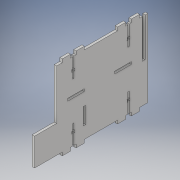
# Autodesk Inventor part: sidewall
Saved by Autodesk Inventor 2018 (Build 220112000, 112)
## iProperties
Created: 2018-03-27
Part Number: sidewall
Material: Generic
Document SubType Name: Modeling
Designer: guita
Density: 1 g/cm^3
Appearance: Default
Author: guita
Autodesk Inventor part; units mm, degrees
ref_plane "YZ Plane" through (0, 0, 0) normal (1, 0, 0) x (0, 1, 0)
ref_plane "XZ Plane" through (0, 0, 0) normal (0, 1, 0) x (-1, 0, 0)
ref_plane "XY Plane" through (0, 0, 0) normal (0, 0, 1) x (1, 0, 0)
sketch "Sketch1" plane through (0, 0, 0) normal (1, 0, 0) x (0, 1, 0)
  line L0 (0, 0) -> (177.8, 0)
  line L1 (177.8, -260.35) -> (0, -260.35)
  line L2 (0, -260.35) -> (0, -241.3)
  line L3 (0, -241.3) -> (-7.62, -241.3)
  line L4 (-7.62, -241.3) -> (-7.62, -222.25)
  line L5 (-7.62, -222.25) -> (0, -222.25)
  line L6 (0, -209.55) -> (-7.62, -209.55)
  line L7 (-7.62, -209.55) -> (-7.62, -190.5)
  line L8 (-7.62, -190.5) -> (0, -190.5)
  line L9 (0, -190.5) -> (0, -152.4)
  line L10 (44.45, -215.9) -> (44.45, -214.2998)
  line L11 (44.45, -217.5002) -> (44.45, -215.9)
  line L12 (24.6348, -214.2998) -> (24.6348, -212.725)
  line L13 (24.6348, -219.075) -> (24.6348, -219.329)
  line L14 (24.6348, -219.329) -> (30.1625, -219.329)
  line L15 (24.6348, -212.725) -> (24.6348, -212.471)
  line L16 (24.6348, -212.471) -> (30.1625, -212.471)
  line L17 (24.6348, -219.075) -> (24.6348, -217.4875)
  line L18 (30.1625, -212.471) -> (30.1625, -214.2998)
  line L19 (30.1625, -217.5002) -> (30.1625, -219.329)
  line L20 (44.45, -214.2998) -> (30.1625, -214.2998)
  line L21 (24.6348, -214.2998) -> (0, -214.2998)
  line L22 (44.45, -217.5002) -> (30.1625, -217.5002)
  line L23 (24.6348, -217.5002) -> (0, -217.5002)
  line L24 (0, -63.5) -> (-7.62, -63.5)
  line L25 (-7.62, -63.5) -> (-7.62, -82.55)
  line L26 (-7.62, -82.55) -> (0, -82.55)
  line L27 (0, -95.25) -> (-7.62, -95.25)
  line L28 (-7.62, -95.25) -> (-7.62, -114.3)
  line L29 (-7.62, -114.3) -> (0, -114.3)
  line L30 (44.45, -88.9) -> (44.45, -90.5002)
  line L31 (44.45, -87.2998) -> (44.45, -88.9)
  line L32 (24.6348, -90.5002) -> (24.6348, -92.075)
  line L33 (24.6348, -85.725) -> (24.6348, -85.471)
  line L34 (24.6348, -85.471) -> (30.1625, -85.471)
  line L35 (24.6348, -92.075) -> (24.6348, -92.329)
  line L36 (24.6348, -92.329) -> (30.1625, -92.329)
  line L37 (24.6348, -85.725) -> (24.6348, -87.3125)
  line L38 (30.1625, -92.329) -> (30.1625, -90.5002)
  line L39 (30.1625, -87.2998) -> (30.1625, -85.471)
  line L40 (44.45, -90.5002) -> (30.1625, -90.5002)
  line L41 (24.6348, -90.5002) -> (0, -90.5002)
  line L42 (44.45, -87.2998) -> (30.1625, -87.2998)
  line L43 (24.6348, -87.2998) -> (0, -87.2998)
  line L44 (177.8, -241.3) -> (185.42, -241.3)
  line L45 (185.42, -241.3) -> (185.42, -222.25)
  line L46 (185.42, -222.25) -> (177.8, -222.25)
  line L47 (177.8, -209.55) -> (185.42, -209.55)
  line L48 (185.42, -209.55) -> (185.42, -190.5)
  line L49 (185.42, -190.5) -> (177.8, -190.5)
  line L50 (177.8, -190.5) -> (177.8, -152.4)
  line L51 (133.35, -215.9) -> (133.35, -214.2998)
  line L52 (133.35, -217.5002) -> (133.35, -215.9)
  line L53 (153.1652, -214.2998) -> (153.1652, -212.725)
  line L54 (153.1652, -219.075) -> (153.1652, -219.329)
  line L55 (153.1652, -219.329) -> (147.6375, -219.329)
  line L56 (153.1652, -212.725) -> (153.1652, -212.471)
  line L57 (153.1652, -212.471) -> (147.6375, -212.471)
  line L58 (153.1652, -219.075) -> (153.1652, -217.4875)
  line L59 (147.6375, -212.471) -> (147.6375, -214.2998)
  line L60 (147.6375, -217.5002) -> (147.6375, -219.329)
  line L61 (133.35, -214.2998) -> (147.6375, -214.2998)
  line L62 (153.1652, -214.2998) -> (177.8, -214.2998)
  line L63 (133.35, -217.5002) -> (147.6375, -217.5002)
  line L64 (153.1652, -217.5002) -> (177.8, -217.5002)
  line L65 (185.42, -63.5) -> (185.42, -82.55)
  line L66 (185.42, -82.55) -> (177.8, -82.55)
  line L67 (177.8, -95.25) -> (185.42, -95.25)
  line L68 (185.42, -95.25) -> (185.42, -114.3)
  line L69 (185.42, -114.3) -> (177.8, -114.3)
  line L70 (153.1652, -85.725) -> (153.1652, -85.471)
  line L71 (153.1652, -85.725) -> (153.1652, -87.3125)
  line L72 (153.1652, -85.471) -> (147.6375, -85.471)
  line L73 (147.6375, -87.2998) -> (147.6375, -85.471)
  line L74 (177.8, -63.5) -> (185.42, -63.5)
  line L75 (153.1652, -90.5002) -> (153.1652, -92.075)
  line L76 (153.1652, -92.075) -> (153.1652, -92.329)
  line L77 (153.1652, -92.329) -> (147.6375, -92.329)
  line L78 (147.6375, -92.329) -> (147.6375, -90.5002)
  line L79 (133.35, -87.2998) -> (147.6375, -87.2998)
  line L80 (133.35, -87.2998) -> (133.35, -88.9)
  line L81 (133.35, -90.5002) -> (147.6375, -90.5002)
  line L82 (153.1652, -87.2998) -> (177.8, -87.2998)
  line L83 (153.1652, -90.5002) -> (177.8, -90.5002)
  line L84 (133.35, -88.9) -> (133.35, -90.5002)
  line L85 (177.8, -260.35) -> (177.8, -254)
  line L86 (177.8, -254) -> (88.9, -254)
  line L87 (88.9, -254) -> (88.9, -247.65)
  line L88 (88.9, -247.65) -> (177.8, -247.65)
  line L89 (177.8, -254) -> (177.8, -260.35)
  line L90 (177.8, 0) -> (177.8, -63.5)
  line L91 (177.8, -114.3) -> (177.8, -190.5)
  line L92 (177.8, -241.3) -> (177.8, -247.65)
  line L93 (0, -260.35) -> (0, -241.3)
  line L94 (0, -190.5) -> (0, -114.3)
  line L95 (0, -63.5) -> (0, 0)
  line L96 (0, -82.55) -> (0, -87.2998)
  line L97 (0, -90.5002) -> (0, -95.25)
  line L98 (0, -95.25) -> (0, -90.5002)
  line L99 (0, -87.2998) -> (0, -82.55)
  line L100 (0, -222.25) -> (0, -217.5002)
  line L101 (0, -214.2998) -> (0, -209.55)
  line L102 (0, -222.25) -> (0, -217.5002)
  line L103 (0, -214.2998) -> (0, -209.55)
  line L104 (177.8, -222.25) -> (177.8, -217.5002)
  line L105 (177.8, -214.2998) -> (177.8, -209.55)
  line L106 (177.8, -209.55) -> (177.8, -214.2998)
  line L107 (177.8, -217.5002) -> (177.8, -222.25)
  line L108 (177.8, -82.55) -> (177.8, -87.2998)
  line L109 (177.8, -90.5002) -> (177.8, -95.25)
  line L110 (177.8, -82.55) -> (177.8, -87.2998)
  line L111 (177.8, -90.5002) -> (177.8, -95.25)
  dimension "d0" = 177.8
  dimension "d1" = 260.35
  dimension "d8" = 38.1
  dimension "d16" = 0.254
  dimension "d17" = 0.254
  dimension "d18" = 6.35
  constraints: 224 end point, 8 point on line, 1 midpoint
  measures "d0" distance of L1.start L1.end
  measures "d1" distance of L0.end L1.start
  measures "d8" distance of L8.end L9.end
  measures "d16" distance of L13.start L13.end
  measures "d17" distance of L12.end L15.end
  measures "d18" distance of L1.start L85.end
extrude "Extrusion1" add sketch "Sketch1" along normal blind 5.5563
sketch "Sketch2" plane through (5.5563, 0, 0) normal (1, 0, 0) x (0, 0, -1)
  line L0 (63.5, 177.8) -> (0, 177.8) projected
  line L1 (0, 177.8) -> (50.8, 177.8)
  line L2 (50.8, 177.8) -> (50.8, 63.5)
  line L3 (50.8, 63.5) -> (0, 63.5)
  line L4 (0, 177.8) -> (0, 0) projected
  line L5 (0, 177.8) -> (0, 63.5)
  constraints: 8 end point, 2 perpendicular, 2 point on line, 1 vertical
extrude "Extrusion2" cut sketch "Sketch2" against normal blind 25.4
sketch "Sketch3" plane through (5.5563, 0, 0) normal (1, 0, 0) x (0, 0, -1)
  line L0 (190.5, 177.8) -> (114.3, 177.8) projected
  line L1 (247.65, 88.9) -> (247.65, 177.8) projected
  line L2 (76.2, 100.8) -> (76.2, 95.25)
  line L3 (114.3, 95.25) -> (114.3, 100.8)
  line L4 (184.15, 100.8) -> (184.15, 95.25)
  line L5 (222.25, 95.25) -> (222.25, 100.8)
  line L6 (76.2, 100.8) -> (114.3, 100.8)
  line L7 (184.15, 100.8) -> (222.25, 100.8)
  line L8 (95.25, 95.25) -> (76.2, 95.25)
  line L9 (95.25, 95.25) -> (114.3, 95.25)
  line L10 (184.15, 95.25) -> (222.25, 95.25)
  point P0 (0, 0)
  constraints: 18 end point, 8 perpendicular, 2 horizontal, 1 point on line, 1 vertical
extrude "Extrusion3" cut sketch "Sketch3" against normal blind 25.4
sketch "Sketch4" plane through (5.5563, 0, 0) normal (1, 0, 0) x (0, 0, -1)
  line L0 (111.9187, 28.194) -> (117.475, 28.194)
  line L1 (117.475, 28.194) -> (117.475, 66.294)
  line L2 (117.475, 66.294) -> (111.9187, 66.294)
  line L3 (111.9187, 47.244) -> (111.9187, 66.294)
  line L4 (111.9187, 28.194) -> (111.9187, 47.244)
  point P0 (0, 0)
  constraints: 10 end point, 3 perpendicular, 1 collinear, 1 point on line
extrude "Extrusion4" cut sketch "Sketch4" against normal blind 25.4
body "Solid1"
